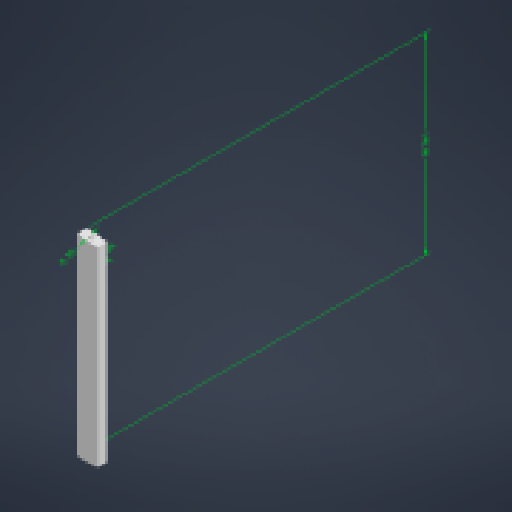
# Autodesk Inventor part: stand2
Saved by Autodesk Inventor 2026.2 (Build 302298000, 298)
## iProperties
Created: 2026-02-23
Part Number: stand2
Material: Generic
Document SubType Name: Modeling
Designer: danda
Density: 1 g/cm^3
Appearance: Default
Author: danda
Autodesk Inventor part; units mm, degrees
ref_plane "YZ Plane" through (0, 0, 0) normal (1, 0, 0) x (0, 1, 0)
ref_plane "XZ Plane" through (0, 0, 0) normal (0, 1, 0) x (-1, 0, 0)
ref_plane "XY Plane" through (0, 0, 0) normal (0, 0, 1) x (1, 0, 0)
sketch "Sketch1" plane through (0, 0, 0) normal (0, 0, 1) x (1, 0, 0)
  line L0 (12.1296, 191.2771) -> (12.1296, 1.2771)
  line L1 (12.1296, 1.2771) -> (32.1296, 1.2771)
  line L2 (12.1296, 191.2771) -> (32.1296, 189.5273)
  line L3 (12.1296, 191.2771) -> (39.6219, 191.2771) construction
  line L4 (32.1296, 1.2771) -> (32.1296, 189.5273)
  point P0 (0, 0)
  dimension "d0" = 190
  dimension "d1" = 20
  dimension "d2" = 5
  constraints: 10 end point, 2 vertical, 1 horizontal, 1 perpendicular
  measures "d0" distance of L0.start L0.end
  measures "d1" distance of L0.end L1.end
  measures "d2" angle of L2 L3
extrude "Extrusion1" add sketch "Sketch1" along normal mid plane 10
sketch "Sketch2" plane through (12.1296, 191.2771, 5) normal (0.0871557, 0.9961947, 0) x (0.9961947, -0.0871557, 0)
  circle A0 centre (9.4291, 5) radius 2.5
  point P0 (4.5875, 5)
  dimension "d7" = 5
  constraints: 1 centre point
  measures "d7" diameter of A0
extrude "Extrusion2" add sketch "Sketch2" along normal blind 2
body "Solid1"
